Autodesk Fusion 360 part; units mm, degrees
(part 2 of 2)
sketch "ToasterText" plane through (0, 0, -1.25) normal (0, 0, -1) x (1, 0, 0) in component "Backplate"
  line L0 (27.7657, -16.7089) -> (28.4378, -16.7089)
  line L1 (28.4378, -16.7089) -> (28.4378, -15.2642)
  spline S0 degree 3 poles (28.4378, -15.2642) (28.4378, -15.1584) (28.4148, -15.0843) (28.369, -15.042) knots 0 0 0 0 1 1 1 1
  spline S1 degree 3 poles (28.369, -15.042) (28.3231, -14.9996) (28.2438, -14.9785) (28.1309, -14.9785) knots 0 0 0 0 1 1 1 1
  spline S2 degree 3 poles (28.1309, -14.9785) (28.018, -14.9785) (27.8892, -14.9944) (27.7446, -15.0261) knots 0 0 0 0 1 1 1 1
  line L2 (27.7446, -15.0261) -> (27.7446, -14.5551)
  spline S3 degree 3 poles (27.7446, -14.5551) (27.9139, -14.5022) (28.0885, -14.4758) (28.2684, -14.4758) knots 0 0 0 0 1 1 1 1
  spline S4 degree 3 poles (28.2684, -14.4758) (28.5295, -14.4758) (28.7209, -14.5322) (28.8426, -14.6451) knots 0 0 0 0 1 1 1 1
  spline S5 degree 3 poles (28.8426, -14.6451) (28.9643, -14.758) (29.0252, -14.9538) (29.0252, -15.2325) knots 0 0 0 0 1 1 1 1
  line L3 (29.0252, -15.2325) -> (29.0252, -16.7089)
  line L4 (29.0252, -16.7089) -> (29.3903, -16.7089)
  line L5 (29.3903, -16.7089) -> (29.3903, -17.1904)
  line L6 (29.3903, -17.1904) -> (29.0093, -17.1904)
  line L7 (29.0093, -17.1904) -> (28.9669, -17.9524)
  line L8 (28.9669, -17.9524) -> (28.4378, -17.9524)
  line L9 (28.4378, -17.9524) -> (28.4378, -17.1904)
  line L10 (28.4378, -17.1904) -> (27.7657, -17.1904)
  line L11 (27.7657, -17.1904) -> (27.7657, -16.7089)
  spline S6 degree 3 poles (27.3689, -16.8941) (27.1572, -17.134) (26.8432, -17.2539) (26.4269, -17.2539) knots 0 0 0 0 1 1 1 1
  spline S7 degree 3 poles (26.4269, -17.2539) (26.0107, -17.2539) (25.6976, -17.134) (25.4877, -16.8941) knots 0 0 0 0 1 1 1 1
  spline S8 degree 3 poles (25.4877, -16.8941) (25.2778, -16.6542) (25.1728, -16.3102) (25.1728, -15.8622) knots 0 0 0 0 1 1 1 1
  line L12 (25.1728, -15.8622) -> (25.1728, -15.8516)
  spline S9 degree 3 poles (25.1728, -15.8516) (25.1728, -15.4036) (25.2778, -15.0587) (25.4877, -14.8171) knots 0 0 0 0 1 1 1 1
  spline S10 degree 3 poles (25.4877, -14.8171) (25.6976, -14.5754) (26.0107, -14.4546) (26.4269, -14.4546) knots 0 0 0 0 1 1 1 1
  spline S11 degree 3 poles (26.4269, -14.4546) (26.8432, -14.4546) (27.1563, -14.5754) (27.3662, -14.8171) knots 0 0 0 0 1 1 1 1
  spline S12 degree 3 poles (27.3662, -14.8171) (27.5761, -15.0587) (27.6811, -15.4036) (27.6811, -15.8516) knots 0 0 0 0 1 1 1 1
  line L13 (27.6811, -15.8516) -> (27.6811, -15.8622)
  spline S13 degree 3 poles (27.6811, -15.8622) (27.6811, -16.3102) (27.577, -16.6542) (27.3689, -16.8941) knots 0 0 0 0 1 1 1 1
  spline S14 degree 3 poles (26.4269, -14.9467) (25.986, -14.9467) (25.7655, -15.2484) (25.7655, -15.8516) knots 0 0 0 0 1 1 1 1
  line L14 (25.7655, -15.8516) -> (25.7655, -15.8622)
  spline S15 degree 3 poles (25.7655, -15.8622) (25.7655, -16.4619) (25.986, -16.7618) (26.4269, -16.7618) knots 0 0 0 0 1 1 1 1
  spline S16 degree 3 poles (26.4269, -16.7618) (26.8644, -16.7618) (27.0831, -16.4619) (27.0831, -15.8622) knots 0 0 0 0 1 1 1 1
  line L15 (27.0831, -15.8622) -> (27.0831, -15.8516)
  spline S17 degree 3 poles (27.0831, -15.8516) (27.0831, -15.2484) (26.8644, -14.9467) (26.4269, -14.9467) knots 0 0 0 0 1 1 1 1
  line L16 (23.2996, -15.55) -> (23.2996, -15.7616)
  line L17 (23.2996, -15.7616) -> (23.7547, -15.7193)
  spline S18 degree 3 poles (23.7547, -15.7193) (24.0122, -15.6946) (24.1974, -15.6532) (24.3103, -15.595) knots 0 0 0 0 1 1 1 1
  spline S19 degree 3 poles (24.3103, -15.595) (24.4232, -15.5368) (24.4796, -15.43) (24.4796, -15.2748) knots 0 0 0 0 1 1 1 1
  line L18 (24.4796, -15.2748) -> (24.4796, -15.2642)
  spline S20 degree 3 poles (24.4796, -15.2642) (24.4796, -15.1513) (24.4435, -15.0649) (24.3711, -15.0049) knots 0 0 0 0 1 1 1 1
  spline S21 degree 3 poles (24.3711, -15.0049) (24.2988, -14.945) (24.1992, -14.915) (24.0722, -14.915) knots 0 0 0 0 1 1 1 1
  spline S22 degree 3 poles (24.0722, -14.915) (23.8393, -14.915) (23.6523, -14.9758) (23.5112, -15.0975) knots 0 0 0 0 1 1 1 1
  spline S23 degree 3 poles (23.5112, -15.0975) (23.3701, -15.2193) (23.2996, -15.3701) (23.2996, -15.55) knots 0 0 0 0 1 1 1 1
  line L19 (24.342, -16.3914) -> (24.9188, -16.3914)
  spline S24 degree 3 poles (24.9188, -16.3914) (24.9082, -16.663) (24.8086, -16.8738) (24.6198, -17.0237) knots 0 0 0 0 1 1 1 1
  spline S25 degree 3 poles (24.6198, -17.0237) (24.4311, -17.1736) (24.1515, -17.2486) (23.7811, -17.2486) knots 0 0 0 0 1 1 1 1
  spline S26 degree 3 poles (23.7811, -17.2486) (23.0756, -17.2486) (22.7228, -16.9523) (22.7228, -16.3596) knots 0 0 0 0 1 1 1 1
  line L20 (22.7228, -16.3596) -> (22.7228, -14.5234)
  line L21 (22.7228, -14.5234) -> (23.2572, -14.5234)
  line L22 (23.2572, -14.5234) -> (23.2731, -14.8991)
  line L23 (23.2731, -14.8991) -> (23.2837, -14.8991)
  spline S27 degree 3 poles (23.2837, -14.8991) (23.3578, -14.7686) (23.4733, -14.6627) (23.6303, -14.5816) knots 0 0 0 0 1 1 1 1
  spline S28 degree 3 poles (23.6303, -14.5816) (23.7873, -14.5005) (23.9681, -14.4599) (24.1727, -14.4599) knots 0 0 0 0 1 1 1 1
  spline S29 degree 3 poles (24.1727, -14.4599) (24.4408, -14.4599) (24.6551, -14.5234) (24.8156, -14.6504) knots 0 0 0 0 1 1 1 1
  spline S30 degree 3 poles (24.8156, -14.6504) (24.9761, -14.7774) (25.0564, -14.9714) (25.0564, -15.2325) knots 0 0 0 0 1 1 1 1
  line L24 (25.0564, -15.2325) -> (25.0564, -15.2431)
  spline S31 degree 3 poles (25.0564, -15.2431) (25.0564, -15.3771) (25.0344, -15.4935) (24.9903, -15.5923) knots 0 0 0 0 1 1 1 1
  spline S32 degree 3 poles (24.9903, -15.5923) (24.9462, -15.6911) (24.8888, -15.7705) (24.8183, -15.8304) knots 0 0 0 0 1 1 1 1
  spline S33 degree 3 poles (24.8183, -15.8304) (24.7477, -15.8904) (24.656, -15.9398) (24.5431, -15.9786) knots 0 0 0 0 1 1 1 1
  spline S34 degree 3 poles (24.5431, -15.9786) (24.4302, -16.0174) (24.3209, -16.0456) (24.215, -16.0633) knots 0 0 0 0 1 1 1 1
  spline S35 degree 3 poles (24.215, -16.0633) (24.1092, -16.0809) (23.9822, -16.0968) (23.834, -16.1109) knots 0 0 0 0 1 1 1 1
  line L25 (23.834, -16.1109) -> (23.3049, -16.1585)
  line L26 (23.3049, -16.1585) -> (23.3049, -16.3596)
  spline S36 degree 3 poles (23.3049, -16.3596) (23.3049, -16.5007) (23.3401, -16.6057) (23.4107, -16.6745) knots 0 0 0 0 1 1 1 1
  spline S37 degree 3 poles (23.4107, -16.6745) (23.4812, -16.7433) (23.6047, -16.7776) (23.7811, -16.7776) knots 0 0 0 0 1 1 1 1
  spline S38 degree 3 poles (23.7811, -16.7776) (24.1409, -16.7776) (24.3279, -16.6489) (24.342, -16.3914) knots 0 0 0 0 1 1 1 1
  spline S39 degree 3 poles (21.3364, -14.9256) (20.9836, -14.9256) (20.8072, -15.0402) (20.8072, -15.2695) knots 0 0 0 0 1 1 1 1
  line L27 (20.8072, -15.2695) -> (20.8072, -15.2801)
  spline S40 degree 3 poles (20.8072, -15.2801) (20.8072, -15.3789) (20.846, -15.4547) (20.9236, -15.5076) knots 0 0 0 0 1 1 1 1
  spline S41 degree 3 poles (20.9236, -15.5076) (21.0012, -15.5606) (21.1212, -15.5976) (21.2834, -15.6188) knots 0 0 0 0 1 1 1 1
  line L28 (21.2834, -15.6188) -> (21.5427, -15.6505)
  spline S42 degree 3 poles (21.5427, -15.6505) (21.8497, -15.6858) (22.0798, -15.7643) (22.2333, -15.886) knots 0 0 0 0 1 1 1 1
  spline S43 degree 3 poles (22.2333, -15.886) (22.3868, -16.0077) (22.4635, -16.1991) (22.4635, -16.4601) knots 0 0 0 0 1 1 1 1
  line L29 (22.4635, -16.4601) -> (22.4635, -16.4707)
  spline S44 degree 3 poles (22.4635, -16.4707) (22.4635, -16.7247) (22.3726, -16.9188) (22.191, -17.0528) knots 0 0 0 0 1 1 1 1
  spline S45 degree 3 poles (22.191, -17.0528) (22.0093, -17.1869) (21.7403, -17.2539) (21.384, -17.2539) knots 0 0 0 0 1 1 1 1
  spline S46 degree 3 poles (21.384, -17.2539) (20.689, -17.2539) (20.3239, -16.984) (20.2886, -16.4443) knots 0 0 0 0 1 1 1 1
  line L30 (20.2886, -16.4443) -> (20.8601, -16.4443)
  spline S47 degree 3 poles (20.8601, -16.4443) (20.8672, -16.5677) (20.913, -16.6559) (20.9977, -16.7089) knots 0 0 0 0 1 1 1 1
  spline S48 degree 3 poles (20.9977, -16.7089) (21.0824, -16.7618) (21.2111, -16.7882) (21.384, -16.7882) knots 0 0 0 0 1 1 1 1
  spline S49 degree 3 poles (21.384, -16.7882) (21.7227, -16.7882) (21.892, -16.6859) (21.892, -16.4813) knots 0 0 0 0 1 1 1 1
  line L31 (21.892, -16.4813) -> (21.892, -16.4707)
  spline S50 degree 3 poles (21.892, -16.4707) (21.892, -16.372) (21.8532, -16.297) (21.7756, -16.2458) knots 0 0 0 0 1 1 1 1
  spline S51 degree 3 poles (21.7756, -16.2458) (21.698, -16.1947) (21.571, -16.1585) (21.3946, -16.1374) knots 0 0 0 0 1 1 1 1
  line L32 (21.3946, -16.1374) -> (21.1512, -16.1056)
  spline S52 degree 3 poles (21.1512, -16.1056) (20.8337, -16.0597) (20.6017, -15.976) (20.4553, -15.8543) knots 0 0 0 0 1 1 1 1
  spline S53 degree 3 poles (20.4553, -15.8543) (20.3089, -15.7325) (20.2357, -15.5394) (20.2357, -15.2748) knots 0 0 0 0 1 1 1 1
  line L33 (20.2357, -15.2748) -> (20.2357, -15.2642)
  spline S54 degree 3 poles (20.2357, -15.2642) (20.2357, -14.7245) (20.6079, -14.4546) (21.3522, -14.4546) knots 0 0 0 0 1 1 1 1
  spline S55 degree 3 poles (21.3522, -14.4546) (22.1248, -14.4546) (22.5182, -14.7474) (22.5323, -15.333) knots 0 0 0 0 1 1 1 1
  line L34 (22.5323, -15.333) -> (21.9555, -15.333)
  spline S56 degree 3 poles (21.9555, -15.333) (21.9484, -15.199) (21.8893, -15.0975) (21.7782, -15.0288) knots 0 0 0 0 1 1 1 1
  spline S57 degree 3 poles (21.7782, -15.0288) (21.6671, -14.96) (21.5198, -14.9256) (21.3364, -14.9256) knots 0 0 0 0 1 1 1 1
  line L35 (18.5529, -16.7089) -> (19.225, -16.7089)
  line L36 (19.225, -16.7089) -> (19.225, -15.2642)
  spline S58 degree 3 poles (19.225, -15.2642) (19.225, -15.1584) (19.2021, -15.0843) (19.1562, -15.042) knots 0 0 0 0 1 1 1 1
  spline S59 degree 3 poles (19.1562, -15.042) (19.1103, -14.9996) (19.031, -14.9785) (18.9181, -14.9785) knots 0 0 0 0 1 1 1 1
  spline S60 degree 3 poles (18.9181, -14.9785) (18.8052, -14.9785) (18.6764, -14.9944) (18.5318, -15.0261) knots 0 0 0 0 1 1 1 1
  line L37 (18.5318, -15.0261) -> (18.5318, -14.5551)
  spline S61 degree 3 poles (18.5318, -14.5551) (18.7011, -14.5022) (18.8757, -14.4758) (19.0557, -14.4758) knots 0 0 0 0 1 1 1 1
  spline S62 degree 3 poles (19.0557, -14.4758) (19.3167, -14.4758) (19.5081, -14.5322) (19.6298, -14.6451) knots 0 0 0 0 1 1 1 1
  spline S63 degree 3 poles (19.6298, -14.6451) (19.7515, -14.758) (19.8124, -14.9538) (19.8124, -15.2325) knots 0 0 0 0 1 1 1 1
  line L38 (19.8124, -15.2325) -> (19.8124, -16.7089)
  line L39 (19.8124, -16.7089) -> (20.1775, -16.7089)
  line L40 (20.1775, -16.7089) -> (20.1775, -17.1904)
  line L41 (20.1775, -17.1904) -> (19.7965, -17.1904)
  line L42 (19.7965, -17.1904) -> (19.7542, -17.9524)
  line L43 (19.7542, -17.9524) -> (19.225, -17.9524)
  line L44 (19.225, -17.9524) -> (19.225, -17.1904)
  line L45 (19.225, -17.1904) -> (18.5529, -17.1904)
  line L46 (18.5529, -17.1904) -> (18.5529, -16.7089)
  spline S64 degree 3 poles (17.0395, -14.9361) (16.7855, -14.9361) (16.5033, -14.9908) (16.1929, -15.1002) knots 0 0 0 0 1 1 1 1
  line L47 (16.1929, -15.1002) -> (16.1929, -14.6239)
  spline S65 degree 3 poles (16.1929, -14.6239) (16.468, -14.5111) (16.7644, -14.4546) (17.0819, -14.4546) knots 0 0 0 0 1 1 1 1
  spline S66 degree 3 poles (17.0819, -14.4546) (17.5652, -14.4546) (17.9179, -14.571) (18.1402, -14.8039) knots 0 0 0 0 1 1 1 1
  spline S67 degree 3 poles (18.1402, -14.8039) (18.3624, -15.0367) (18.4736, -15.3859) (18.4736, -15.8516) knots 0 0 0 0 1 1 1 1
  line L48 (18.4736, -15.8516) -> (18.4736, -15.8622)
  spline S68 degree 3 poles (18.4736, -15.8622) (18.4736, -16.3067) (18.366, -16.6498) (18.1508, -16.8914) knots 0 0 0 0 1 1 1 1
  spline S69 degree 3 poles (18.1508, -16.8914) (17.9356, -17.1331) (17.6216, -17.2539) (17.2089, -17.2539) knots 0 0 0 0 1 1 1 1
  spline S70 degree 3 poles (17.2089, -17.2539) (16.4398, -17.2539) (16.0553, -16.8323) (16.0553, -15.9892) knots 0 0 0 0 1 1 1 1
  spline S71 degree 3 poles (16.0553, -15.9892) (16.0553, -15.8904) (16.0659, -15.774) (16.087, -15.6399) knots 0 0 0 0 1 1 1 1
  line L49 (16.087, -15.6399) -> (17.9021, -15.6399)
  spline S72 degree 3 poles (17.9021, -15.6399) (17.895, -15.3965) (17.8236, -15.2184) (17.6878, -15.1055) knots 0 0 0 0 1 1 1 1
  spline S73 degree 3 poles (17.6878, -15.1055) (17.5519, -14.9926) (17.3359, -14.9361) (17.0395, -14.9361) knots 0 0 0 0 1 1 1 1
  spline S74 degree 3 poles (16.7485, -16.6083) (16.8367, -16.7283) (16.9919, -16.7882) (17.2142, -16.7882) knots 0 0 0 0 1 1 1 1
  spline S75 degree 3 poles (17.2142, -16.7882) (17.4364, -16.7882) (17.6022, -16.7291) (17.7116, -16.611) knots 0 0 0 0 1 1 1 1
  spline S76 degree 3 poles (17.7116, -16.611) (17.8209, -16.4928) (17.8844, -16.3102) (17.9021, -16.0633) knots 0 0 0 0 1 1 1 1
  line L50 (17.9021, -16.0633) -> (16.6109, -16.0633)
  spline S77 degree 3 poles (16.6109, -16.0633) (16.6144, -16.3102) (16.6603, -16.4919) (16.7485, -16.6083) knots 0 0 0 0 1 1 1 1
  line L51 (15.8224, -14.5234) -> (15.8224, -17.1904)
  line L52 (15.8224, -17.1904) -> (15.2457, -17.1904)
  line L53 (15.2457, -17.1904) -> (15.2351, -16.6983)
  line L54 (15.2351, -16.6983) -> (15.2245, -16.6983)
  spline S78 degree 3 poles (15.2245, -16.6983) (15.1716, -16.8606) (15.0754, -16.9964) (14.9361, -17.1057) knots 0 0 0 0 1 1 1 1
  spline S79 degree 3 poles (14.9361, -17.1057) (14.7967, -17.2151) (14.6054, -17.261) (14.3619, -17.2433) knots 0 0 0 0 1 1 1 1
  line L55 (14.3619, -17.2433) -> (14.3619, -16.6612)
  spline S80 degree 3 poles (14.3619, -16.6612) (14.6724, -16.6612) (14.8955, -16.5969) (15.0313, -16.4681) knots 0 0 0 0 1 1 1 1
  spline S81 degree 3 poles (15.0313, -16.4681) (15.1672, -16.3393) (15.2351, -16.1268) (15.2351, -15.8304) knots 0 0 0 0 1 1 1 1
  line L56 (15.2351, -15.8304) -> (15.2351, -14.5234)
  line L57 (15.2351, -14.5234) -> (15.8224, -14.5234)
  arc A0 (29.1775, -20.325) -> (31.4275, -18.075) centre (29.1775, -18.075) ccw
  line L58 (31.4275, -18.075) -> (31.4275, -14.575)
  arc A1 (31.4275, -14.575) -> (29.1775, -12.325) centre (29.1775, -14.575) ccw
  line L59 (29.1775, -12.325) -> (14.6775, -12.325)
  arc A2 (14.6775, -12.325) -> (12.4275, -14.575) centre (14.6775, -14.575) ccw
  line L60 (12.4275, -14.575) -> (12.4275, -18.075)
  arc A3 (12.4275, -18.075) -> (14.6775, -20.325) centre (14.6775, -18.075) ccw
  line L61 (14.6775, -20.325) -> (29.1775, -20.325)
extrude "Extrude10" add sketch "ToasterText" along normal blind 0.25 contours L0 L1 S0 S1 S2 L2 S3 S4 S5 L3 L4 L5 L6 L7 L8 L9 L10 L11 | S6 S7 S8 L12 S9 S10 S11 S12 L13 S13 | L19 S24 S25 S26 L20 L21 L22 L23 S27 S28 S29 S30 L24 S31 S32 S33 S34 S35 L25 L26 S36 S37 S38 | S39 L27 S40 S41 L28 S42 S43 L29 S44 S45 S46 L30 S47 S48 S49 L31 S50 S51 L32 S52 S53 L33 S54 S55 L34 S56 S57 | L35 L36 S58 S59 S60 L37 S61 S62 S63 L38 L39 L40 L41 L42 L43 L44 L45 L46 | S64 L47 S65 S66 S67 L48 S68 S69 S70 S71 L49 S72 S73 | L51 L52 L53 L54 S78 S79 L55 S80 S81 L56 L57 bodies 8 in component "Backplate"
fillet "Fillet6" radius 0.1 13 edges at (29.0093, 17.1904, -1.375) (28.4378, 17.1904, -1.375) (29.0252, 16.7089, -1.375) (28.4378, 16.7089, -1.375) (23.2996, 15.7616, -1.375) (23.2731, 14.8991, -1.375) (19.7965, 17.1904, -1.375) (19.225, 17.1904, -1.375) (19.8124, 16.7089, -1.375) (19.225, 16.7089, -1.375) (17.9021, 16.0633, -1.375) (16.6109, 16.0633, -1.375) (15.2351, 16.6983, -1.375) on bodies 8 in component "Backplate"
sketch "Board (2)" plane through (0, 0, 0) normal (0, 0, 1) x (1, 0, 0) in component "Board"
  line L0 (4.75, 0) -> (39.105, 0)
  arc A0 (0, 4.75) -> (4.75, 0) centre (4.75, 4.75) ccw
  line L1 (0, 27.9) -> (0, 4.75)
  line L2 (41.5, 27.94) -> (41.5, 32.002)
  arc A1 (39.105, 0) -> (43.855, 4.75) centre (39.105, 4.75) ccw
  arc A2 (41.5, 32.002) -> (39.105, 32.65) centre (39.105, 27.9) ccw
  line L3 (39.105, 32.65) -> (4.75, 32.65)
  arc A3 (4.75, 32.65) -> (0, 27.9) centre (4.75, 27.9) ccw
  line L4 (43.855, 4.75) -> (43.855, 27.94)
  line L5 (41.5, 27.94) -> (43.855, 27.94)
  arc A4 (1.6764, 7.5345) -> (1.6764, 8.8095) centre (1.6764, 8.172) ccw
  arc A5 (41.9, 18.0295) -> (41.9, 16.7545) centre (41.9, 17.392) ccw
  arc A6 (41.9, 16.7545) -> (41.9, 18.0295) centre (41.9, 17.392) ccw
  arc A7 (1.6764, 8.8095) -> (1.6764, 7.5345) centre (1.6764, 8.172) ccw
  arc A8 (1.6764, 8.8095) -> (1.6764, 7.5345) centre (1.6764, 8.172) ccw
  arc A9 (41.9, 18.0295) -> (41.9, 16.7545) centre (41.9, 17.392) ccw
  arc A10 (41.9, 16.7545) -> (41.9, 18.0295) centre (41.9, 17.392) ccw
  arc A11 (41.9, 18.0295) -> (41.9, 16.7545) centre (41.9, 17.392) ccw
  arc A12 (1.94, 29.0375) -> (1.94, 27.7625) centre (1.94, 28.4) ccw
  arc A13 (1.6764, 8.8095) -> (1.6764, 7.5345) centre (1.6764, 8.172) ccw
  arc A14 (1.6764, 7.5345) -> (1.6764, 8.8095) centre (1.6764, 8.172) ccw
  arc A15 (1.94, 27.7625) -> (1.94, 29.0375) centre (1.94, 28.4) ccw
  arc A16 (1.94, 29.0375) -> (1.94, 27.7625) centre (1.94, 28.4) ccw
  arc A17 (1.6764, 8.8095) -> (1.6764, 7.5345) centre (1.6764, 8.172) ccw
  arc A18 (1.94, 27.7625) -> (1.94, 29.0375) centre (1.94, 28.4) ccw
  arc A19 (41.9, 18.0295) -> (41.9, 16.7545) centre (41.9, 17.392) ccw
  arc A20 (41.9, 16.7545) -> (41.9, 18.0295) centre (41.9, 17.392) ccw
  arc A21 (41.9, 16.7545) -> (41.9, 18.0295) centre (41.9, 17.392) ccw
  arc A22 (1.6764, 7.5345) -> (1.6764, 8.8095) centre (1.6764, 8.172) ccw
  arc A23 (1.94, 29.0375) -> (1.94, 27.7625) centre (1.94, 28.4) ccw
  arc A24 (1.94, 27.7625) -> (1.94, 29.0375) centre (1.94, 28.4) ccw
  arc A25 (1.94, 27.7625) -> (1.94, 29.0375) centre (1.94, 28.4) ccw
  arc A26 (1.94, 29.0375) -> (1.94, 27.7625) centre (1.94, 28.4) ccw
  arc A27 (1.6764, 7.5345) -> (1.6764, 8.8095) centre (1.6764, 8.172) ccw
  arc A28 (1.94, 29.0692) -> (1.94, 27.7308) centre (1.94, 28.4) ccw
  arc A29 (1.6764, 8.8413) -> (1.6764, 7.5028) centre (1.6764, 8.172) ccw
  arc A30 (1.94, 27.7308) -> (1.94, 29.0692) centre (1.94, 28.4) ccw
  arc A31 (41.9, 18.0612) -> (41.9, 16.7228) centre (41.9, 17.392) ccw
  arc A32 (1.6764, 7.5028) -> (1.6764, 8.8413) centre (1.6764, 8.172) ccw
  arc A33 (41.9, 16.7228) -> (41.9, 18.0612) centre (41.9, 17.392) ccw
  arc A34 (1.94, 27.7308) -> (1.94, 29.0692) centre (1.94, 28.4) ccw
  arc A35 (41.9, 18.0612) -> (41.9, 16.7228) centre (41.9, 17.392) ccw
  arc A36 (1.6764, 8.8413) -> (1.6764, 7.5028) centre (1.6764, 8.172) ccw
  arc A37 (1.94, 29.0692) -> (1.94, 27.7308) centre (1.94, 28.4) ccw
  arc A38 (41.9, 16.7228) -> (41.9, 18.0612) centre (41.9, 17.392) ccw
  arc A39 (1.6764, 7.5028) -> (1.6764, 8.8413) centre (1.6764, 8.172) ccw
  point P0 (1.6764, 8.172)
  point P1 (41.9, 17.392)
  point P2 (1.94, 28.4)
extrude "Board" add sketch "Board (2)" along normal blind 3.1 separate body contours L0 A0 L1 L2 A1 A2 L3 A3 L4 L5 makes body 9 in component "Board"
move_body "Board (1)" bodies 9 to x (1, 0, 0) y (0, 1, 0) z (0, 0, 1) at (0, 0, 11.2) in component "Board"
sketch "Sketch1" plane through (0, 0, 0) normal (0, 0, 1) x (1, 0, 0) in component "Battery"
  line L0 (20, 15) -> (-20, 15)
  line L1 (-20, 15) -> (-20, -15)
  line L2 (-20, -15) -> (20, -15)
  line L3 (20, -15) -> (20, 15)
  line L4 (20, 15) -> (-20, -15) construction
  dimension "d443" = 40
  dimension "d444" = 30
  constraint horizontal L0
  constraint vertical L1
  constraint horizontal L2
  constraint vertical L3
  constraint midpoint L4 origin
  measures "d443" distance of L1 L3
  measures "d444" distance of L0 L2
extrude "Extrude1'" add sketch "Sketch1" along normal blind 11.2 separate body makes body 10 in component "Battery"
move_body "Align1'" bodies 10 to x (1, 0, 0) y (0, 1, 0) z (0, 0, 1) at (21.9275, 16.325, 0) in component "Battery"
component "Front" placed x (1, 0, 0) y (0, 1, 0) z (0, 0, 1) at (0, 0, 0)
component "Button" placed x (1, 0, 0) y (0, 1, 0) z (0, 0, 1) at (0, 0, 0)
component "Backplate" placed x (1, 0, 0) y (0, 1, 0) z (0, 0, 1) at (0, 0, 0)
component "Board" placed x (1, 0, 0) y (0, 1, 0) z (0, 0, 1) at (0, 0, 0)
component "Battery" placed x (1, 0, 0) y (0, 1, 0) z (0, 0, 1) at (0, 0, 0)
equation "BoardHeight = 32.65 mm"
equation "BoardWidth = 43.855 mm"
equation "EnclosureThickness = 1.5 mm"
equation "ImageSensorX = 33.5424 mm"
equation "ImageSensorY = 17.392 mm"
equation "MotionSensorX = 7.5 mm"
equation "MotionSensorY = 17.392 mm"
equation "MotionSensorDiameter = 9.3 mm + 0.5 mm + EnclosureMfgTol"
equation "LensProtrusionOutsideThickness = 13.5287 mm + 2 mm"
equation "LensProtrusionDepth = LensThreadDepth - MountPointDepth"
equation "OuterEdgeRadius = 6 mm"
equation "BoardRadius = 4.75 mm"
equation "MountPoint2X = 1.682 mm"
equation "MountPoint2Y = 8.172 mm"
equation "MountPointDepth = USBCReceptacleWidth + 0.3 mm"
equation "MountPoint3X = 41.9 mm"
equation "MountPoint3Y = 19 mm"
equation "MountPoint1X = 1.94 mm"
equation "MountPoint1Y = 28.4 mm"
equation "BackplateMountPointDepth = EnclosureDepth"
equation "BackplateMountPointWidth = 1.5 mm"
equation "HoleDiameter = 10 mm"
equation "BatteryWidth = 40 mm"
equation "BatteryHeight = 30 mm"
equation "BatteryThickness = 11 mm + 0.2 mm"
equation "BackplateOverlap = 0.2 mm"
equation "BackplateHoleOffset = ( BackplateMountPointWidth - EnclosureThickness ) / 2"
equation "ScrewHeadDiameter = 3 mm"
equation "ScrewHeadHeight = 1 mm"
equation "BackplateThickness = 1.5 mm"
equation "EnclosureDepth = FrontplateThickness + MountPointDepth + BoardThickness + BatteryThickness"
equation "BoardThickness = 3.1 mm"
equation "BoardEnclosureGap = 0.15 mm"
equation "USBCReceptacleCutoutWidth = USBCReceptacleWidth + USBCReceptacleTolerance + 2 * EnclosureMfgTol"
equation "USBCReceptacleCutoutHeight = USBCReceptacleHeight + USBCReceptacleTolerance + 2 * EnclosureMfgTol"
equation "USBCReceptacleCutoutRadius = 2.4 mm / 2 - 0.2 mm"
equation "USBCReceptacleY = 5.25348125 mm"
equation "USBCReceptacleWidth = 3.16 mm"
equation "d329 = BoardWidth"
equation "d330 = BoardHeight"
equation "d331 = BoardRadius"
equation "d332 = BoardEnclosureGap"
equation "d333 = EnclosureThickness"
equation "d334 = EnclosureDepth"
equation "d336 = BoardEnclosureGap + BackplateOverlap"
equation "d337 = BoardEnclosureGap + BackplateOverlap + BackplateGap"
equation "d350 = MotionSensorX"
equation "d351 = MotionSensorY"
equation "d352 = ImageSensorX"
equation "d353 = ImageSensorY"
equation "d354 = FrontplateThickness"
equation "MountPointHeight = 3 mm"
equation "MountPointRadius = 1.5 mm"
equation "d443 = BatteryWidth"
equation "d444 = BatteryHeight"
equation "d445 = BatteryThickness"
equation "d492 = USBCReceptacleCutoutWidth"
equation "d493 = USBCReceptacleCutoutHeight"
equation "d497 = USBCReceptacleCutoutRadius"
equation "d498 = USBCReceptacleCutoutRadius"
equation "d499 = USBCReceptacleCutoutRadius"
equation "d502 = EnclosureMfgTol"
equation "d505 = -USBCReceptacleY"
equation "USBCReceptacleHeight = 8.94 mm"
equation "USBCReceptacleTolerance = 0.2 mm"
equation "EnclosureMfgTol = 0.1 mm"
equation "FrontplateThickness = 4.3 mm"
equation "LensThreadDepth = 9.2 mm" comment "Lens threaded region length + lens back focal length (BFL)"
equation "LensProtrusionInsideThickness = 13.0287 mm + 2 mm"
equation "d540 = -MountPointDepth"
equation "d542 = -MountPointDepth"
equation "d544 = LensProtrusionDepth"
equation "d546 = LensProtrusionDepth"
equation "d554 = LensProtrusionInsideThickness"
equation "d555 = LensProtrusionOutsideThickness"
equation "BackplateDovetailAngle = 10 deg"
equation "d575 = LensOringOutsideDiameter"
equation "LensOringOutsideDiameter = 13.5 mm + 0.1 mm"
equation "LensOringThickness = 1 mm"
equation "LensOringSeatDepth = 0.5 mm"
equation "d590 = MountPointDepth"
equation "d592 = MountPointDepth"
equation "d594 = LensProtrusionBoardGap"
equation "d596 = -MountPointDepth"
equation "LensProtrusionBoardGap = 0.25 mm" comment "Gap between inside lens protrusion and board"
equation "d598 = -MountPointDepth + LensProtrusionBoardGap"
equation "d599 = LensOringSeatDepth"
equation "d601 = -MountPointDepth"
equation "d602 = LensProtrusionBoardGap"
equation "d604 = MountPointHoleDepth"
equation "d611 = -MountPointDepth"
equation "MountPointHoleDepth = 2.6 mm"
equation "DovetailAngle = 10 deg"
equation "DovetailFillet = 0.5 mm"
equation "d641 = FrontplateFillet"
equation "FrontplateFillet = 2 mm"
equation "TextEngraveDepth = 0.25 mm"
equation "d647 = ImageSensorX"
equation "d648 = LEDY"
equation "d649 = FrontplateThickness"
equation "d650 = LEDHoleDiameter"
equation "LEDHoleDiameter = 0.75 mm"
equation "d653 = BoardThickness"
equation "d662 = MountPointHeight"
equation "d663 = MountPoint1Width"
equation "d664 = MountPoint2Width"
equation "d665 = MountPointHeight"
equation "d666 = MountPointHeight"
equation "d667 = MountPoint3Width"
equation "d668 = MountPoint2X"
equation "d669 = MountPoint2Y"
equation "d670 = MountPoint1X"
equation "d671 = MountPoint1Y"
equation "d672 = MountPoint3Y"
equation "d673 = MountPoint3X"
equation "BackplateIndentAngle = 10 deg"
equation "BackplateIndentOffset = 17 mm"
equation "BackplateGap = 0.075 mm"
equation "BackplateIndentRadius = 1 mm"
equation "BackplateIndentWidth = 5 mm"
equation "BackplateIndentHeight = 8 mm"
equation "BackplateIndentDepth = 0.5 mm"
equation "d762 = MountPointRadius"
equation "d763 = ButtonY"
equation "d764 = ImageSensorX"
equation "ButtonY = 4.75 mm"
equation "LEDY = 28.8 mm"
equation "ButtonDiameter = 3 mm"
equation "ButtonHoleDiameter = ButtonDiameter + ButtonEnclosureClearance"
equation "d771 = FrontplateThickness"
equation "d772 = ButtonHoleDiameter"
equation "d774 = ButtonDiameter"
equation "ButtonProtrusion = 0.6 mm"
equation "ButtonHeight = MountPointDepth + FrontplateThickness + ButtonProtrusion - TactileSwitchHeight"
equation "TactileSwitchHeight = 0.6 mm + 0.1 mm"
equation "d785 = ButtonHeight"
equation "d789 = ButtonProtrusion"
equation "d790 = ButtonHoleDiameter"
equation "ButtonStopperHeight = MountPointDepth - TactileSwitchHeight"
equation "ButtonStopperDiameter = 3.6 mm"
equation "ButtonEnclosureClearance = 0.2 mm"
equation "d794 = ButtonStopperDiameter"
equation "d795 = ButtonStopperHeight"
equation "BackplateMountPointHeight = 3 mm"
equation "d809 = BackplateMountPointY"
equation "BackplateMountPointY = BoardHeight / 2"
equation "d812 = BackplateMountPointWidth"
equation "d813 = MountPointHeight"
equation "d814 = BackplateMountPointY"
equation "d815 = BackplateMountPointDepth"
equation "d819 = BackplateMountPointWidth"
equation "d820 = MountPointHeight"
equation "d821 = BackplateMountPointY"
equation "d822 = MountPointHoleDepth"
equation "d825 = BackplateHoleOffset"
equation "d826 = BackplateHoleOffset"
equation "MountPoint1Width = 3 mm"
equation "MountPoint2Width = 3 mm"
equation "MountPoint3Width = 5 mm"
equation "d857 = EnclosureThickness"
equation "d858 = BackplateThickness"
equation "d860 = BackplateThickness"
equation "d862 = BackplateThickness"
equation "d872 = -TextEngraveDepth"
equation "d874 = BackplateEngravingRectWidth"
equation "d875 = BackplateEngravingRectHeight"
equation "d876 = BackplateEngravingRectRadius"
equation "BackplateEngravingRectRadius = 2.25 mm"
equation "BackplateEngravingRectWidth = 19 mm"
equation "BackplateEngravingRectHeight = 8 mm"
equation "d880 = -TextEngraveDepth"
equation "d882 = TextEngraveDepth"
equation "d888 = MotionSensorRadius1"
equation "MotionSensorRadius1 = 11 mm + MotionSensorTolerance"
equation "MotionSensorRadius2 = 10.4 mm + MotionSensorTolerance"
equation "MotionSensorRadius3 = 9.3 mm + MotionSensorTolerance"
equation "MotionSensorRadius4 = 9 mm + MotionSensorTolerance"
equation "d896 = -MotionSensorMidpointOffset"
equation "d897 = MotionSensorRadius2"
equation "d898 = MotionSensorRadius3"
equation "d899 = -MotionSensorEndpointOffset"
equation "d900 = MotionSensorRadius4"
equation "MotionSensorTolerance = 0.25 mm" comment "Datasheet says tolerance is 0.5, but that's substantial, so we went with half that"
equation "MotionSensorMidpointOffset = 5.8 mm + MotionSensorTolerance"
equation "MotionSensorEndpointOffset = 9.9 mm"
equation "BoardCutoutRadius = 2 * BackplateMountPointWidth + 0.2 mm"
equation "d905 = BoardCutoutRadius"
equation "BoardCutoutTriWidth = 1.5 mm"
equation "BoardCutoutTriHeight = 4.5 mm"
equation "d911 = BoardCutoutTriHeight"
equation "d912 = BoardCutoutTriWidth"
named bodies: "Body", "Front", "USBCPlugCutout", "BackplateMountPoint1", "BackplateMountPoint2", "MotionSensor"
